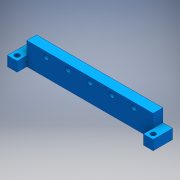
# Autodesk Inventor part: frameBottomRight
Saved by Autodesk Inventor 2016 (Build 200138000, 138)
## iProperties
Created: 2016-05-25
Part Number: frameBottomRight
Material: ABS Plastic
Document SubType Name: Modeling
Designer: Henrik Samuelsson
Density: 1.06 g/cm^3
Appearance: Smooth - White
Author: Henrik Samuelsson
Autodesk Inventor part; units mm, degrees
ref_plane "YZ Plane" through (0, 0, 0) normal (1, 0, 0) x (0, 1, 0)
ref_plane "XZ Plane" through (0, 0, 0) normal (0, 1, 0) x (-1, 0, 0)
ref_plane "XY Plane" through (0, 0, 0) normal (0, 0, 1) x (1, 0, 0)
sketch "Sketch1" plane through (0, 0, 0) normal (0, 1, 0) x (-1, 0, 0)
  line L0 (0, 0) -> (-180, 0)
  line L1 (-180, 0) -> (-180, -12)
  line L2 (-180, -12) -> (0, -12)
  line L3 (0, -12) -> (0, 0)
  line L4 (-90, 0) -> (-90, 10)
  circle A0 centre (-90, 10) radius 3
  circle A1 centre (-117, 10) radius 3
  circle A2 centre (-144, 10) radius 3
  circle A3 centre (-63, 10) radius 3
  circle A4 centre (-36, 10) radius 3
  line L5 (-12, 0) -> (-12, 16)
  line L6 (-12, 16) -> (-168, 16)
  line L7 (-168, 16) -> (-168, 0)
  line L8 (0, 0) -> (-12, 0)
  line L9 (-168, 0) -> (-180, 0)
  dimension "d0" = 180
  dimension "d1" = 12
  dimension "d2" = 10
  dimension "d3" = 6
  dimension "d4" = 6
  dimension "d5" = 6
  dimension "d7" = 6
  dimension "d8" = 6
  dimension "d10" = 27
  dimension "d11" = 27
  dimension "d13" = 27
  dimension "d14" = 27
  dimension "d16" = 10
  dimension "d17" = 10
  dimension "d18" = 10
  dimension "d19" = 10
  dimension "d20" = 12
  dimension "d21" = 12
  dimension "d22" = 6
  constraints: 20 end point, 5 centre point, 4 perpendicular, 2 collinear, 2 parallel, 2 point on line, 1 coincident, 1 horizontal, 1 midpoint, 1 vertical
  measures "d0" distance of L2.end L1.end
  measures "d1" distance of L1.end L0.end
  measures "d2" distance of L4.start L4.end
  measures "d3" diameter of A0
  measures "d4" diameter of A1
  measures "d5" diameter of A2
  measures "d7" diameter of A3
  measures "d8" diameter of A4
  measures "d10" distance of A3.centre L4.end
  measures "d11" distance of A4.centre A3.centre
  measures "d13" distance of A1.centre L4.end
  measures "d14" distance of A1.centre A2.centre
  measures "d16" distance from line of L0 A4.centre
  measures "d17" distance from line of L0 A3.centre
  measures "d18" distance from line of L0 A1.centre
  measures "d19" distance from line of L0 A2.centre
  measures "d20" distance of L0.start L5.start
  measures "d21" distance of L7.end L0.end
  measures "d22" distance from line of L6 A4.centre
extrude "Extrusion1" add sketch "Sketch1" along normal blind 12
sketch "Sketch2" plane through (0, 0, 0) normal (0, -1, 0) x (1, 0, 0)
  line L0 (0, 0) -> (12, 0)
  line L1 (12, 0) -> (12, -12)
  line L2 (12, -12) -> (0, -12)
  line L3 (0, -12) -> (0, 0)
  line L4 (180, 0) -> (180, -12) projected
  line L5 (168, 0) -> (180, 0) projected
  line L6 (180, -12) -> (168, -12)
  line L7 (168, -12) -> (168, 0)
  line L8 (168, 0) -> (180, 0)
  line L9 (180, 0) -> (180, -12)
  dimension "d25" = 12
  dimension "d26" = 12
  constraints: 16 end point, 4 parallel, 2 horizontal, 2 perpendicular
  measures "d25" distance of L1.end L2.end
  measures "d26" distance of L0.end L1.end
extrude "Extrusion2" add sketch "Sketch2" along normal blind 12
sketch "Sketch3" plane through (180, 12, -12) normal (0, 0, -1) x (-1, 0, 0)
  circle A0 centre (174, -18) radius 3
  circle A1 centre (6, -18) radius 3
  line L0 (168, -12) -> (168, -24) projected
  line L1 (180, -24) -> (168, -24) projected
  line L2 (12, -12) -> (12, -24) projected
  line L3 (12, -24) -> (0, -24) projected
  point P0 (180, -12)
  dimension "d29" = 6
  dimension "d30" = 6
  dimension "d31" = 6
  dimension "d32" = 6
  dimension "d33" = 6
  dimension "d34" = 6
  constraints: 2 centre point
  measures "d29" diameter of A0
  measures "d30" diameter of A1
  measures "d31" distance from line of L0 A0.centre
  measures "d32" distance from line of L1 A0.centre
  measures "d33" distance from line of L2 A1.centre
  measures "d34" distance from line of L3 A1.centre
extrude "Extrusion3" cut sketch "Sketch3" against normal up to next
sketch "Sketch4" plane through (0, 12, 0) normal (0, 1, 0) x (1, 0, 0)
  point P0 (0, 0)
body "Solid1"
